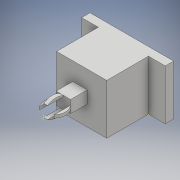
# Autodesk Inventor part: robotarm
Saved by Autodesk Inventor 2018 (Build 220112000, 112)
## iProperties
Created: 2018-01-21
Part Number: robotarm
Material: Generic
Document SubType Name: Modeling
Designer: abdul
Density: 1 g/cm^3
Appearance: Default
Author: abdul
Autodesk Inventor part; units mm, degrees
ref_plane "YZ Plane" through (0, 0, 0) normal (1, 0, 0) x (0, 1, 0)
ref_plane "XZ Plane" through (0, 0, 0) normal (0, 1, 0) x (-1, 0, 0)
ref_plane "XY Plane" through (0, 0, 0) normal (0, 0, 1) x (1, 0, 0)
sketch "Sketch1" plane through (0, 0, 0) normal (0, 0, 1) x (1, 0, 0)
  line L0 (0, 0) -> (100, 0)
  line L1 (100, 0) -> (100, 10)
  line L2 (100, 10) -> (0, 10)
  line L3 (0, 10) -> (0, 0)
  line L4 (20, 0) -> (80, 0)
  line L5 (80, 0) -> (80, -50)
  line L6 (80, -50) -> (20, -50)
  line L7 (20, -50) -> (20, 0)
  dimension "d0" = 100
  dimension "d1" = 10
  dimension "d2" = 60
  dimension "d3" = 50
  constraints: 16 end point, 4 parallel, 2 horizontal, 2 perpendicular, 1 point on line
  measures "d0" distance of L2.end L1.end
  measures "d1" distance of L1.end L0.end
  measures "d2" distance of L5.end L6.end
  measures "d3" distance of L4.end L5.end
extrude "Extrusion1" add sketch "Sketch1" along normal blind 60
sketch "Sketch2" plane through (80, -50, 0) normal (1, 0, 0) x (0, 0, -1)
  point P0 (0, 50)
sketch "Sketch3" plane through (20, -50, 0) normal (0, -1, 0) x (1, 0, 0)
  line L0 (36.7526, 23.8482) -> (19.4451, 23.8482)
  line L1 (19.4451, 23.8482) -> (19.4451, 38.5395)
  line L2 (19.4451, 38.5395) -> (36.7526, 38.5395)
  line L3 (36.7526, 38.5395) -> (36.7526, 23.8482)
  point P0 (-20, 0)
  constraints: 8 end point, 2 parallel, 1 horizontal, 1 perpendicular
extrude "Extrusion2" add sketch "Sketch3" along normal blind 20
sketch "Sketch4" plane through (20, -70, 0) normal (0, -1, 0) x (1, 0, 0)
  line L0 (36.7526, 38.5395) -> (36.7526, 23.8482) projected
  line L1 (36.7526, 29.0807) -> (40.5764, 29.0807)
  line L2 (40.5764, 29.0807) -> (40.5764, 32.502)
  line L3 (40.5764, 32.502) -> (36.7526, 32.502)
  line L4 (36.7526, 32.502) -> (36.7526, 29.0807)
  line L5 (19.4451, 38.5395) -> (19.4451, 23.8482) projected
  line L6 (19.4451, 32.502) -> (16.2251, 32.502)
  line L7 (16.2251, 32.502) -> (16.2251, 29.0807)
  line L8 (16.2251, 29.0807) -> (19.4451, 29.0807)
  line L9 (19.4451, 29.0807) -> (19.4451, 32.502)
  line L10 (19.4451, 38.5395) -> (36.7526, 38.5395) projected
  line L11 (29.3064, 38.5395) -> (24.6776, 38.5395)
  line L12 (24.6776, 38.5395) -> (24.6776, 41.7595)
  line L13 (24.6776, 41.7595) -> (29.3064, 41.7595)
  line L14 (29.3064, 41.7595) -> (29.3064, 38.5395)
  line L15 (36.7526, 23.8482) -> (19.4451, 23.8482) projected
  line L16 (29.3064, 23.8482) -> (24.6776, 23.8482)
  line L17 (24.6776, 23.8482) -> (24.6776, 20.8294)
  line L18 (24.6776, 20.8294) -> (29.3064, 20.8294)
  line L19 (29.3064, 20.8294) -> (29.3064, 23.8482)
  point P0 (-20, 0)
  constraints: 32 end point, 8 parallel, 8 point on line, 4 horizontal, 4 perpendicular
extrude "Extrusion3" add sketch "Sketch4" along normal blind 20 contours L3 L2 L1 L0 | L10 L12 L13 L14 | L19 L18 L17 L15 | L5 L8 L7 L6
sketch "Sketch5" plane through (44.6776, -70, 20.8294) normal (-1, 0, 0) x (0, 0, 1)
  point P0 (-20.8294, 70)
sketch "Sketch6" plane through (44.6776, -70, 20.8294) normal (-1, 0, 0) x (0, 0, 1)
  point P0 (-20.8294, 70)
sketch "Sketch7" plane through (44.6776, -70, 20.8294) normal (-1, 0, 0) x (0, 0, 1)
  point P0 (-20.8294, 70)
  point P1 (3.0188, -20)
sketch "Sketch8" plane through (36.2251, -70, 29.0807) normal (-1, 0, 0) x (0, 0, 1)
  point P0 (-29.0807, 70)
sketch "Sketch9" plane through (60.5764, -70, 29.0807) normal (0, 0, -1) x (-1, 0, 0)
  line L0 (3.8238, 0) -> (3.8238, -20) projected
  arc A0 (3.8238, 0) -> (3.8238, -19.7321) centre (14.64, -9.866) ccw
  line L1 (3.8238, 0) -> (0, 0) projected
  line L2 (3.8238, 0) -> (0, 0)
  line L3 (0, 0) -> (0, -9.866)
  line L4 (0, 0) -> (0, -20) projected
  line L5 (3.8238, -20) -> (0, -20) projected
  line L6 (0, -20) -> (3.8238, -20) projected
  line L7 (0, -20) -> (3.8238, -20)
  point P0 (60.5764, 70)
  constraints: 6 end point, 3 point on circle, 2 horizontal, 2 point on line, 1 centre point
extrude "Extrusion4" cut sketch "Sketch9" against normal blind 20 contours A0 L3 L1 | L0 L5 L4 A0
sketch "Sketch10" plane through (39.4451, -70, 29.0807) normal (0, 0, -1) x (-1, 0, 0)
  line L0 (0, -20) -> (3.22, -20) projected
  line L1 (0, 0) -> (0, -20) projected
  arc A0 (0, -20) -> (0, 0) centre (-13.9179, -10) ccw
  line L2 (0, 0) -> (3.22, 0)
  line L3 (3.22, 0) -> (3.22, -10)
  line L4 (3.22, 0) -> (3.22, -20) projected
  point P0 (39.4451, 70)
  constraints: 4 end point, 2 point on circle, 1 centre point, 1 horizontal, 1 midpoint
extrude "Extrusion5" cut sketch "Sketch10" against normal blind 20 contours A0 L4 L0 | L2 L3 A0
sketch "Sketch11" plane through (44.6776, -70, 20.8294) normal (-1, 0, 0) x (0, 0, 1)
  line L0 (3.0188, 0) -> (3.0188, -20) projected
  arc A0 (3.0188, 0) -> (3.0188, -20) centre (18.0725, -10) ccw
  line L1 (3.0188, 0) -> (0, 0) projected
  line L2 (3.0188, 0) -> (0, 0)
  line L3 (0, 0) -> (0, -10)
  line L4 (0, 0) -> (0, -20) projected
  line L5 (0, -20) -> (3.0188, -20) projected
  line L6 (0, -20) -> (3.0188, -20)
  point P0 (-20.8294, 70)
  constraints: 6 end point, 2 point on circle, 1 centre point, 1 collinear, 1 horizontal, 1 midpoint, 1 point on line
extrude "Extrusion6" cut sketch "Sketch11" against normal blind 20 contours A0 L3 L1 | L5 L4 A0
sketch "Sketch12" plane through (44.6776, -70, 38.5395) normal (-1, 0, 0) x (0, 0, 1)
  line L0 (0, 0) -> (0, -20) projected
  arc A0 (0, -20) -> (0, 0) centre (-13.9179, -10) ccw
  line L1 (-6.0375, 0) -> (0, 0) projected
  line L2 (0, 0) -> (3.22, 0) projected
  line L3 (0, 0) -> (3.22, 0)
  line L4 (3.22, 0) -> (3.22, -10)
  line L5 (3.22, 0) -> (3.22, -20) projected
  line L6 (0, -20) -> (3.22, -20) projected
  line L7 (3.22, -20) -> (0, -20)
  point P0 (-38.5395, 70)
  constraints: 6 end point, 3 point on circle, 1 centre point, 1 collinear, 1 horizontal
extrude "Extrusion7" cut sketch "Sketch12" against normal blind 20 contours L2 L4 A0 | A0 L5 L6
body "Solid1"
